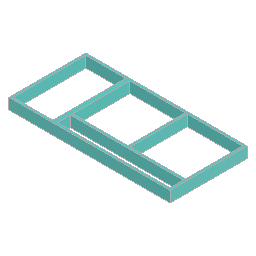
Digital-Storage-Holdster (Autodesk Fusion 360 design; units mm, degrees)
Autodesk Fusion 360 part; units mm, degrees
sketch "Sketch1" plane through (0, 0, 3.175) normal (0, 0, 1) x (-1, 0, 0)
  line L0 (0, 0) -> (0, 297.942)
  line L1 (0, 297.942) -> (-407.924, 297.942)
  line L2 (-407.924, 297.942) -> (-407.924, 0)
  line L3 (-407.924, 0) -> (0, 0)
  line L4 (0, 297.942) -> (-60, 297.942)
  line L5 (-60, 297.942) -> (-60, 192.942)
  line L6 (-60, 192.942) -> (0, 192.942)
  line L7 (0, 192.942) -> (0, 297.942)
  line L8 (-2.95, 294.992) -> (-57.05, 294.992)
  line L9 (-57.05, 294.992) -> (-57.05, 195.892)
  line L10 (-57.05, 195.892) -> (-2.95, 195.892)
  line L11 (-2.95, 195.892) -> (-2.95, 294.992)
  point P0 (0, 297.942)
  dimension "d1" = 60
  dimension "d2" = 105
  constraint horizontal L4
  constraint vertical L5
  constraint horizontal L6
  constraint vertical L7
  constraint coincident P0 L0.end
  measures "d1" distance of P0 L4.end
  measures "d2" distance of P0 L6.end
extrude "Extrude1" add sketch "Sketch1" along normal blind 15 contours L0 L1 L4 L5 L6 L7
sketch "Sketch2" plane through (0, 0, 3.175) normal (0, 0, 1) x (-1, 0, 0)
  line L0 (0, 0) -> (0, 297.942)
  line L1 (0, 297.942) -> (-407.924, 297.942)
  line L2 (-407.924, 297.942) -> (-407.924, 0)
  line L3 (-407.924, 0) -> (0, 0)
  line L4 (-60, 297.942) -> (-220, 297.942)
  line L5 (-220, 297.942) -> (-220, 192.942)
  line L6 (-220, 192.942) -> (-60, 192.942)
  line L7 (-60, 192.942) -> (-60, 297.942)
  line L8 (-63.05, 294.892) -> (-216.95, 294.892)
  line L9 (-63.05, 276.892) -> (-216.95, 276.892)
  line L10 (-216.95, 276.892) -> (-216.95, 294.892)
  line L11 (-216.95, 294.892) -> (-63.05, 294.892)
  line L12 (-63.05, 294.892) -> (-63.05, 276.892)
  line L13 (-63.05, 195.992) -> (-63.05, 273.842)
  line L14 (-63.05, 276.892) -> (-63.05, 294.892)
  line L15 (-216.95, 294.892) -> (-216.95, 276.892)
  line L16 (-216.95, 273.842) -> (-216.95, 195.992)
  line L17 (-141.525, 273.842) -> (-141.525, 195.992)
  line L18 (-138.475, 273.842) -> (-138.475, 195.992)
  line L19 (-216.95, 195.992) -> (-141.525, 195.992)
  line L20 (-138.475, 195.992) -> (-63.05, 195.992)
  line L21 (-63.05, 273.842) -> (-138.475, 273.842)
  line L22 (-141.525, 273.842) -> (-216.95, 273.842)
  point P0 (-60, 297.942)
  dimension "d88" = 160
  dimension "d89" = 105
  dimension "d93" = 153.9
  dimension "d94" = 18
  dimension "d96" = 3.05
  dimension "d126" = 3.05
  dimension "d127" = 3.05
  dimension "d128" = 3.05
  dimension "d129" = 3.05
  dimension "d130" = 3.05
  dimension "d131" = 3.05
  dimension "d135" = 3.05
  dimension "d136" = 3.05
  dimension "d137" = 75.425
  dimension "d138" = 75.425
  constraint horizontal L4
  constraint vertical L5
  constraint horizontal L6
  constraint vertical L7
  constraint coincident P0 L4.start
  constraint horizontal L9
  constraint vertical L10
  constraint horizontal L11
  constraint vertical L12
  constraint coincident L9.start L13
  constraint coincident L8 L11.end
  constraint coincident L16.start L15
  constraint perpendicular L15 L21
  constraint collinear L13 L14
  constraint collinear L15 L16
  constraint collinear L19 L20
  constraint collinear L21 L22
  measures "d88" distance of P0 L4.end
  measures "d89" distance of P0 L6.end
  measures "d93" distance of L9.start L9.end
  measures "d94" distance of L9.start L8.start
  measures "d96" distance of L9 L21
  measures "d126" distance of L4 L11
  measures "d127" distance of L5 L15
  measures "d128" distance of L7 L8.start
  measures "d129" distance of L7 L13.end
  measures "d130" distance of L6 L20
  measures "d131" distance of L6 L17.end
  measures "d135" distance of L9 L21
  measures "d136" distance of L17 L18
  measures "d137" distance of L13.start L18.end
  measures "d138" distance of L16.end L17.end
extrude "Extrude2" add sketch "Sketch2" along normal blind 15 contours L1 L4 L5 L6 L7
equation "d1 = OnlineStorageWidth"
equation "d2 = OnlineStorageLength"
equation "d5 = -HoldersterWallWidth + SmallTolerence"
equation "d9 = HoldersterHeightLow"
equation "d88 = WritingEquipmentWidth"
equation "d89 = WritingEquipmentLength"
equation "d93 = WritingEquipmentPenWidth"
equation "d94 = WritingEquipmentPenLength"
equation "d96 = HoldersterWallWidth + SmallTolerence"
equation "d104 = HoldersterHeightLow"
equation "d126 = HoldersterWallWidth + SmallTolerence"
equation "d127 = HoldersterWallWidth + SmallTolerence"
equation "d129 = HoldersterWallWidth + SmallTolerence"
equation "d130 = HoldersterWallWidth + SmallTolerence"
equation "d131 = HoldersterWallWidth + SmallTolerence"
equation "d136 = HoldersterWallWidth + SmallTolerence"
equation "SmallTolerence = 0.05 mm"
equation "HoldersterWallWidth = 3 mm"
equation "OnlineStorageLength = 105 mm"
equation "OnlineStorageWidth = 60 mm"
equation "HoldersterHeightLow = 15 mm"
equation "WritingEquipmentLength = 105 mm"
equation "WritingEquipmentWidth = 160 mm"
equation "WritingEquipmentPenWidth = 153.9 mm"
equation "WritingEquipmentPenLength = 18 mm"
